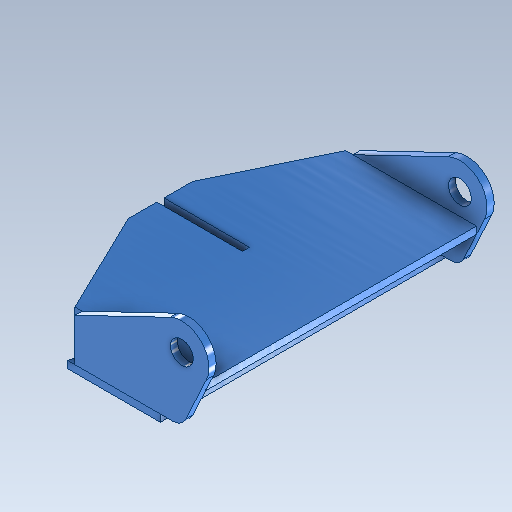
# Autodesk Inventor part: PWTR-0135
Saved by Autodesk Inventor 2021.1 (Build 251245010, 245A)
## iProperties
RuleStatus: InUse
Created: 2020-09-03
Part Number: PWTR-0135
Material: Steel, High Strength, Low Alloy
Document SubType Name: Sheet Metal
Designer: alid
Density: 7.85 g/cm^3
Sheet Metal Rule: Default_mm
Appearance: Cyan
Description: Wheel Bracket
Mass: 1600.01 g
Surface Area: 908.438 cm^2
Volume: 203.823 cm^3
Author: alid
Revision Number: A
Autodesk Inventor part; units mm, degrees
ref_plane "YZ Plane" through (0, 0, 0) normal (1, 0, 0) x (0, 1, 0)
ref_plane "Work Plane1" through (0, 0, 25) normal (0, 0, 1) x (1, 0, 0)
ref_plane "Work Plane2" through (0, -100, 0) normal (0, 1, 0) x (-1, 0, 0)
sketch "LayoutSK" plane through (0, 0, 25) normal (0, 0, 1) x (1, 0, 0)
  circle A0 centre (0, 0) radius 387.5 construction
  line L0 (0, 0) -> (387.5, 0) construction
  line L1 (374.3745, 100) -> (374.3745, -100) construction
  circle A1 centre (0, 0) radius 382.5
  dimension "dia" = 775
  dimension "d17" = 200
  dimension "d28" = 5
  constraints: 4 end point, 3 point on circle, 2 centre point, 1 coincident, 1 horizontal, 1 vertical
  measures "dia" diameter of A0
  measures "d17" distance of L1.start L1.end
  measures "d28" radial gap between concentric circles of A0 A1
sketch "Sketch1" plane through (0, -100, 0) normal (0, 1, 0) x (-1, 0, 0)
  line L0 (-374.3745, 0) -> (-374.3745, 30)
  line L1 (-374.3745, 30) -> (-441.125, 62.1355)
  line L2 (-449.3745, 0) -> (-374.3745, 0)
  line L3 (-449.3745, 0) -> (-466.6105, 36.9627)
  arc A0 (-441.125, 62.1355) -> (-466.6105, 36.9627) centre (-449.3745, 45) ccw
  point P0 (0, 0)
  point P1 (-374.3745, 25)
  point P2 (-374.3745, 25)
  point P3 (-374.3745, 25)
  dimension "d0" = 30
  dimension "d2" = 75
  dimension "d13" = 45
  dimension "d14" = 75
  dimension "d15" = 115
  measures "d0" distance of L0.start L0.end
  measures "d2" distance of L2.start L0.start
  measures "d13" distance from line of A0.centre L2
  measures "d14" distance from line of L0 A0.centre
  measures "d15" angle of L2 L3
extrude "Plate1" add sketch "Sketch1" along normal blind 5
sketch "Sketch2" plane through (0, -100, 0) normal (0, -1, 0) x (1, 0, 0)
  arc A0 (466.6105, 36.9627) -> (441.125, 62.1355) centre (449.3745, 45) ccw projected
  point P0 (0, 0)
  constraints: 1 coincident
hole "Hole1" at (449.3745, -100, 45) direction (0, 1, 0) diameter 16 end through all
mirror "Mirror1" about plane through (0, 0, 0) normal (0, 1, 0)
sketch "Sketch4" plane through (0, 0, 25) normal (0, 0, 1) x (1, 0, 0)
  line L0 (374.3745, -95) -> (461.0322, -95)
  line L1 (461.0322, -95) -> (461.0322, -100)
  line L2 (461.0322, -100) -> (374.3745, -100)
  line L3 (374.3745, 100) -> (461.0322, 100)
  line L4 (461.0322, 100) -> (461.0322, 95)
  line L5 (461.0322, 95) -> (374.3745, 95)
  line L6 (334.3745, 2.5) -> (394.3745, 2.5)
  line L7 (394.3745, 2.5) -> (394.3745, -2.5)
  line L8 (394.3745, -2.5) -> (334.3745, -2.5)
  line L9 (461.0322, 95) -> (461.0322, -95)
  line L10 (334.3745, 2.5) -> (334.3745, 22.5)
  line L11 (334.3745, -2.5) -> (334.3745, -22.5)
  line L12 (374.3745, -100) -> (374.3745, -95)
  line L13 (374.3745, 95) -> (374.3745, 100)
  line L14 (374.3745, 95) -> (369.3745, 95)
  line L15 (374.3745, -95) -> (369.3745, -95)
  line L16 (369.3745, -95) -> (334.3745, -22.5)
  line L17 (334.3745, 22.5) -> (369.3745, 95)
  point P0 (0, 0)
  point P1 (394.3745, 0)
  point P2 (461.0322, 0)
  dimension "d20" = 5
  dimension "d21" = 20
  dimension "d23" = 60
  dimension "d26" = 5
  dimension "d27" = 40
  measures "d20" distance of L6.end L7.end
  measures "d21" distance of L6.start L10.end
  measures "d23" distance of L6.start L6.end
  measures "d26" distance of L5.end L14.end
  measures "d27" distance from line of L5.end L10
extrude "Plate2" add sketch "Sketch4" along normal blind 5 separate body contours L15 L16 L11 L8 L7 L6 L10 L17 L14 L5 L9 L0
sketch "Sketch5" plane through (0, 0, 0) normal (0, 0, 1) x (1, 0, 0)
  line L0 (449.3745, -100) -> (374.3745, -100)
  line L1 (449.3745, 100) -> (374.3745, 100)
  circle A0 centre (0, 0) radius 382.5
  line L2 (449.3745, -100) -> (449.3745, 100)
  line L3 (449.3745, 100) -> (369.1968, 100)
  line L4 (449.3745, -100) -> (369.1968, -100)
  line L5 (434.3745, 100) -> (434.3745, -100)
  point P0 (443.0038, 100)
  dimension "d30" = 15
  measures "d30" distance between parallel lines of L2 L5
extrude "Plate3" add sketch "Sketch5" against normal blind 5 separate body contours L0 L4 A0 L3 L1 L5
fillet "Corner Round1" radius 10 2 edges at (449.3745, -97.5, 0) (449.3745, 97.5, 0)
equation "\"d2\" = d14"
equation "\"d11\" = Thickness"
equation "\"d5\" = Thickness"
equation "\"d24\" = Thickness"
equation "\"d29\" = Thickness"
equation "\"BendRadius\" = Thickness"
equation "\"BendReliefWidth\" = Thickness"
equation "\"BendReliefDepth\" = 0.5 * Thickness"
equation "\"TransitionRadius\" = BendRadius"
equation "\"JacobiRadiusSize\" = BendRadius"
equation "\"GapSize\" = Thickness"
equation "\"Thickness\" = 5"
body "Solid1"
body "Solid2"
body "Solid3"
body "Solid4"
